Autodesk Fusion 360 part; units mm, degrees
(part 2 of 2)
extrude "Extrude53" add sketch "Sketch37" along normal blind 5.5 contours L0 L1 L2 L3 L4 L5 L6 L7 L9 L10 L11 L12 L13 A5 L16 L18 bodies 2
sketch "Sketch38" plane through (0, 10.5, 0) normal (0, 1, 0) x (-1, 0, 0)
  circle A0 centre (-61.5, 36.5) radius 1.75
  circle A1 centre (-61.5, 5.5) radius 1.75
  line L0 (-56, 21) -> (-56, 42)
  line L1 (-56, 42) -> (-56.125, 42)
  line L2 (-56.125, 42) -> (-56.125, 33.4286)
  line L3 (-56.125, 33.4286) -> (-56.125, 30)
  line L4 (-56.125, 30) -> (-58.125, 30)
  line L5 (-58.125, 30) -> (-58.125, 33.4286)
  line L6 (-58.125, 33.4286) -> (-58.125, 42)
  line L7 (-58.125, 42) -> (-67, 42)
  line L8 (-67, 42) -> (-67, 0)
  line L9 (-67, 0) -> (-25, 0)
  line L10 (-25, 0) -> (-25, 42)
  line L11 (-25, 42) -> (-33.875, 42)
  line L12 (-33.875, 42) -> (-33.875, 33.4286)
  line L13 (-33.875, 33.4286) -> (-33.875, 30)
  line L14 (-33.875, 30) -> (-35.875, 30)
  line L15 (-35.875, 30) -> (-35.875, 33.4286)
  line L16 (-35.875, 33.4286) -> (-35.875, 42)
  line L17 (-35.875, 42) -> (-36, 42)
  line L18 (-36, 42) -> (-36, 21)
  arc A2 (-56, 21) -> (-36, 21) centre (-46, 21) ccw
  circle A3 centre (-30.5, 36.5) radius 1.75
  circle A4 centre (-30.5, 5.5) radius 1.75
  line L19 (-33.875, 30) -> (-35.875, 30)
  line L20 (-35.875, 30) -> (-35.875, 42)
  line L21 (-35.875, 42) -> (-33.875, 42)
  line L22 (-33.875, 42) -> (-33.875, 30)
  line L23 (-56.125, 30) -> (-58.125, 30)
  line L24 (-58.125, 30) -> (-58.125, 42)
  line L25 (-58.125, 42) -> (-56.125, 42)
  line L26 (-56.125, 42) -> (-56.125, 30)
  constraint horizontal L19
  constraint vertical L20
  constraint horizontal L21
  constraint vertical L22
  constraint coincident L16.end L17.start
  constraint coincident L13.end L14.start
  constraint horizontal L23
  constraint vertical L24
  constraint horizontal L25
  constraint vertical L26
  constraint coincident L6.end L7.start
  constraint coincident L3.end L4.start
extrude "Extrude54" add sketch "Sketch38" against normal blind 10.5 contours L2 L3 L4 L5 L6 L23 L24 L25 L26 | L12 L13 L14 L15 L16 L19 L20 L21 L22 bodies 2
sketch "Sketch39" plane through (0, 10.5, 0) normal (0, 1, 0) x (-1, 0, 0)
  circle A0 centre (-61.5, 36.5) radius 1.75
  circle A1 centre (-61.5, 5.5) radius 1.75
  line L0 (-56, 21) -> (-56, 42)
  line L1 (-56, 42) -> (-56.125, 42)
  line L2 (-56.125, 42) -> (-56.125, 33.4286)
  line L3 (-56.125, 33.4286) -> (-58.125, 33.4286)
  line L4 (-58.125, 33.4286) -> (-58.125, 42)
  line L5 (-58.125, 42) -> (-67, 42)
  line L6 (-67, 42) -> (-67, 0)
  line L7 (-67, 0) -> (-25, 0)
  line L8 (-25, 0) -> (-25, 42)
  line L9 (-25, 42) -> (-33.875, 42)
  line L10 (-33.875, 42) -> (-33.875, 33.4286)
  line L11 (-33.875, 33.4286) -> (-35.875, 33.4286)
  line L12 (-35.875, 33.4286) -> (-35.875, 42)
  line L13 (-35.875, 42) -> (-36, 42)
  line L14 (-36, 42) -> (-36, 21)
  arc A2 (-56, 21) -> (-36, 21) centre (-46, 21) ccw
  circle A3 centre (-30.5, 36.5) radius 1.75
  circle A4 centre (-30.5, 5.5) radius 1.75
  circle A5 centre (-46, 21) radius 10.125
  line L15 (-46, 21) -> (-35.875, 21)
  line L16 (-35.875, 21) -> (-56.125, 21)
  line L17 (-56.125, 21) -> (-56.125, 42)
  line L18 (-56.125, 42) -> (-35.875, 42)
  line L19 (-35.875, 42) -> (-35.875, 21)
  dimension "d229" = 20.25
  constraint concentric A2 A5
  constraint coincident A2.centre A5.centre
  constraint coincident A5 L15.end
  constraint perpendicular L14 L15
  constraint horizontal L16
  constraint vertical L17
  constraint horizontal L18
  constraint vertical L19
  constraint coincident L1.end L2.start
  measures "d229" diameter of A5
extrude "Extrude55" cut sketch "Sketch39" against normal blind 5.5 contours L0 A5 L16 | A2 A5 L15 L16 | L0 L1 L2 A5 L17 L18 | L0 L14 A5 L18 | L14 A5 L15 L16 | L12 L13 L14 A5 L18 L19 bodies 2
sketch "Sketch40" plane through (0, 0, 42) normal (0, 0, 1) x (1, 0, 0)
  line L0 (67, 0) -> (67, 10.5)
  line L1 (67, 10.5) -> (58.125, 10.5)
  line L2 (58.125, 10.5) -> (58.125, 0)
  line L3 (58.125, 0) -> (67, 0)
  line L4 (67, 5.25) -> (63.5, 5.25)
  circle A0 centre (63.5, 5.25) radius 1.25
  dimension "d232" = 3.5
  dimension "d233" = 2.5
  constraint midpoint L0 L4.start
  constraint perpendicular L0 L4
  constraint coincident L4.end A0.centre
  measures "d232" distance of L4.start L4.end
  measures "d233" diameter of A0
extrude "Extrude56" cut sketch "Sketch40" against normal blind 3 contours A0 bodies 2
sketch "Sketch41" plane through (0, 0, 42) normal (0, 0, 1) x (1, 0, 0)
  line L0 (25, 0) -> (33.875, 0)
  line L1 (33.875, 0) -> (33.875, 10.5)
  line L2 (33.875, 10.5) -> (25, 10.5)
  line L3 (25, 10.5) -> (25, 0)
  line L4 (25, 5.25) -> (28.5, 5.25)
  circle A0 centre (28.5, 5.25) radius 1.25
  dimension "d236" = 3.5
  dimension "d237" = 2.5
  constraint midpoint L3 L4.start
  constraint perpendicular L3 L4
  constraint coincident L4.end A0.centre
  measures "d236" distance of L4.start L4.end
  measures "d237" diameter of A0
extrude "Extrude57" cut sketch "Sketch41" against normal blind 3 contours A0 bodies 2
sketch "Sketch42" plane through (0, 0, 0) normal (0, 0, -1) x (-1, 0, 0)
  line L0 (-67, 0) -> (-25, 0)
  line L1 (-25, 0) -> (-25, 10.5)
  line L2 (-25, 10.5) -> (-67, 10.5)
  line L3 (-67, 10.5) -> (-67, 0)
  line L4 (-67, 5.25) -> (-63.5, 5.25)
  circle A0 centre (-63.5, 5.25) radius 1.25
  line L5 (-25, 5.25) -> (-28.5, 5.25)
  circle A1 centre (-28.5, 5.25) radius 1.25
  dimension "d240" = 3.5
  dimension "d241" = 2.5
  dimension "d242" = 3.5
  dimension "d243" = 2.5
  constraint midpoint L3 L4.start
  constraint perpendicular L3 L4
  constraint coincident L4.end A0.centre
  constraint midpoint L1 L5.start
  constraint perpendicular L1 L5
  constraint coincident L5.end A1.centre
  measures "d240" distance of L4.start L4.end
  measures "d241" diameter of A0
  measures "d242" distance of L5.start L5.end
  measures "d243" diameter of A1
extrude "Extrude58" cut sketch "Sketch42" against normal blind 3 contours A0 | A1 bodies 2
sketch "Sketch43" plane through (0, 0, 42) normal (0, 0, -1) x (-1, 0, 0)
  line L0 (-35.875, 22.25) -> (-35.875, 24.25)
  line L1 (-35.875, 24.25) -> (-56.125, 24.25)
  line L2 (-56.125, 24.25) -> (-56.125, 22.25)
  line L3 (-56.125, 22.25) -> (-48.5, 22.25)
  line L4 (-48.5, 22.25) -> (-48.5, 15.95)
  line L5 (-48.5, 15.95) -> (-43.5, 15.95)
  line L6 (-43.5, 15.95) -> (-43.5, 22.25)
  line L7 (-43.5, 22.25) -> (-35.875, 22.25)
  line L8 (-48.5, 24.25) -> (-43.5, 24.25)
  line L9 (-43.5, 24.25) -> (-43.5, 5)
  line L10 (-43.5, 5) -> (-48.5, 5)
  line L11 (-48.5, 5) -> (-48.5, 24.25)
  dimension "d246" = 19.25
  constraint horizontal L8
  constraint vertical L9
  constraint horizontal L10
  constraint vertical L11
  constraint coincident L1 L8.start
  measures "d246" distance of L8.start L10.end
extrude "Extrude59" add sketch "Sketch43" along normal blind 5 contours L1 L4 L5 L6 L8 L9 L11 | L5 L9 L10 L11 bodies 2
sketch "Sketch44" plane through (43.5, 0, 0) normal (-1, 0, 0) x (0, 0, 1)
  line L0 (52, 22.25) -> (42, 22.25)
  line L1 (42, 22.25) -> (42, 24.25)
  line L2 (42, 24.25) -> (37, 24.25)
  line L3 (37, 24.25) -> (37, 5)
  line L4 (37, 5) -> (42, 5)
  line L5 (42, 5) -> (42, 2)
  line L6 (42, 2) -> (52, 2)
  line L7 (52, 2) -> (52, 8.34)
  line L8 (52, 8.34) -> (42, 8.34)
  line L9 (42, 8.34) -> (42, 15.95)
  line L10 (42, 15.95) -> (52, 15.95)
  line L11 (52, 15.95) -> (52, 22.25)
  line L12 (42, 24.25) -> (37, 5)
  constraint coincident L1.end L2.start
  constraint coincident L3.end L4.start
extrude "Extrude60" cut sketch "Sketch44" against normal blind 12.625 contours L2 L3 L12 bodies 2
extrude "Extrude61" cut 1 faces at (46.0249, 15.95, 43.3343) along direction (0, 1, 0) blind 0.25 on bodies 2 bodies 2
extrude "Extrude62" add 1 faces at (38.2537, 24.25, 47.0497) along direction (0, 1, 0) blind 0.5 on bodies 2 bodies 2
extrude "Extrude63" cut 1 faces at (40.9583, 22.25, 45.3333) along direction (0, 1, 0) blind 0.25 on bodies 2 bodies 2
extrude "Extrude64" cut 1 faces at (51.0417, 22.25, 45.3333) along direction (0, 1, 0) blind 0.25 on bodies 2 bodies 2
extrude "Extrude65" cut 1 faces at (48.5, 5.1133, 48.6667) along direction (-1, 0, 0) blind 0.125 on bodies 2 bodies 2
extrude "Extrude66" cut 1 faces at (43.5, 5.1133, 48.6667) along direction (1, 0, 0) blind 0.125 on bodies 2 bodies 2
sketch "Sketch45" plane through (43.625, 0, 0) normal (-1, 0, 0) x (0, 0, 1)
  line L0 (42, 16.2) -> (52, 16.2)
  line L1 (52, 16.2) -> (52, 22.5)
  line L2 (52, 22.5) -> (42, 22.5)
  line L3 (42, 22.5) -> (42, 24.25)
  line L4 (42, 24.25) -> (37, 5)
  line L5 (37, 5) -> (42, 5)
  line L6 (42, 5) -> (42, 2)
  line L7 (42, 2) -> (52, 2)
  line L8 (52, 2) -> (52, 8.34)
  line L9 (52, 8.34) -> (42, 8.34)
  line L10 (42, 8.34) -> (42, 16.2)
  line L11 (42, 24.25) -> (42, 24.75)
  line L12 (42, 24.75) -> (33, 5)
  line L13 (33, 5) -> (37, 5)
  constraint coincident L3.end L4.start
  constraint parallel L3 L11
  constraint coincident L4.end L5.start
extrude "Extrude67" add sketch "Sketch45" against normal blind 4.75 contours L4 L11 L12 L13 bodies 2
extrude "Extrude68" cut 1 faces at (45.7478, 10.5, 6.5076) along direction (0, -1, 0) blind 10.5 on bodies 2 bodies 2
sketch "Sketch46" plane through (0, 5, 0) normal (0, 1, 0) x (-1, 0, 0)
  line L0 (-48.375, 33) -> (-48.375, 42)
  line L1 (-48.375, 42) -> (-56.125, 42)
  line L2 (-56.125, 42) -> (-56.125, 33.4286)
  line L3 (-56.125, 33.4286) -> (-56.125, 21)
  arc A0 (-56.125, 21) -> (-35.875, 21) centre (-46, 21) ccw
  line L4 (-35.875, 21) -> (-35.875, 33.4286)
  line L5 (-35.875, 33.4286) -> (-35.875, 42)
  line L6 (-35.875, 42) -> (-43.625, 42)
  line L7 (-43.625, 42) -> (-43.625, 33)
  line L8 (-43.625, 33) -> (-48.375, 33)
  circle A1 centre (-46, 21) radius 8.625
  line L9 (-34, 42) -> (-61, 42)
  line L10 (-61, 42) -> (-61, 10)
  line L11 (-61, 10) -> (-34, 10)
  line L12 (-34, 10) -> (-34, 42)
  constraint horizontal L9
  constraint vertical L10
  constraint horizontal L11
  constraint vertical L12
extrude "Extrude69" cut sketch "Sketch46" along normal blind 41 and the other way blind 18 bodies 2
sketch "Sketch47" plane through (33.875, 0, 0) normal (-1, 0, 0) x (0, 0, 1)
  line L0 (33.4286, 10.5) -> (33.4286, 0)
  line L1 (33.4286, 0) -> (52, 0)
  line L2 (52, 0) -> (52, 24.75)
  line L3 (52, 24.75) -> (42, 24.75)
  line L4 (42, 24.75) -> (42, 24.25)
  line L5 (42, 24.25) -> (33.4286, 10.5)
  line L6 (42, 0) -> (42, 24.75)
  line L7 (42, 0) -> (27, 0)
  line L8 (27, 0) -> (27, 26)
  line L9 (27, 26) -> (42, 26)
  line L10 (42, 26) -> (42, 0)
  constraint coincident L1 L6.start
  constraint coincident L3.end L4.start
  constraint horizontal L7
  constraint vertical L8
  constraint horizontal L9
  constraint vertical L10
extrude "Extrude70" cut sketch "Sketch47" against normal blind 10 contours L0 L1 L5 L6 L7 L10 bodies 2
sketch "Sketch48" plane through (0, 0, 42) normal (0, 0, -1) x (-1, 0, 0)
  line L0 (-33.875, 0) -> (-33.875, 24.75)
  line L1 (-33.875, 24.75) -> (-58.125, 24.75)
  line L2 (-58.125, 24.75) -> (-58.125, 0)
  line L3 (-58.125, 0) -> (-33.875, 0)
  line L4 (-48.375, 16.2) -> (-43.625, 16.2)
  line L5 (-43.625, 16.2) -> (-43.625, 22.5)
  line L6 (-43.625, 22.5) -> (-35.875, 22.5)
  line L7 (-35.875, 22.5) -> (-35.875, 2)
  line L8 (-35.875, 2) -> (-43.625, 2)
  line L9 (-43.625, 2) -> (-43.625, 8.34)
  line L10 (-43.625, 8.34) -> (-48.375, 8.34)
  line L11 (-48.375, 8.34) -> (-48.375, 2)
  line L12 (-48.375, 2) -> (-56.125, 2)
  line L13 (-56.125, 2) -> (-56.125, 22.5)
  line L14 (-56.125, 22.5) -> (-48.375, 22.5)
  line L15 (-48.375, 22.5) -> (-48.375, 16.2)
  line L16 (-56.125, 22.5) -> (-56.125, 19)
  line L17 (-56.125, 19) -> (-35.875, 19)
  line L18 (-56.125, 2) -> (-56.125, 5.5)
  line L19 (-56.125, 5.5) -> (-35.875, 5.5)
  line L20 (-56.125, 19) -> (-55, 19)
  line L21 (-55, 19) -> (-55, 5.5)
  line L22 (-35.875, 5.5) -> (-37, 5.5)
  line L23 (-37, 5.5) -> (-37, 19)
  constraint coincident L13.end L14.start
  constraint coincident L13 L16.end
  constraint perpendicular L14 L16
  constraint coincident L7 L17.end
  constraint perpendicular L7 L17
  constraint coincident L12.end L13.start
  constraint coincident L13 L18.end
  constraint perpendicular L12 L18
  constraint coincident L7 L19.end
  constraint perpendicular L7 L19
  constraint coincident L17 L20.end
  constraint perpendicular L16 L20
  constraint coincident L19 L21.end
  constraint perpendicular L19 L21
  constraint coincident L19 L22.end
  constraint perpendicular L7 L22
  constraint coincident L17 L23.end
  constraint perpendicular L17 L23
extrude "Extrude71" add sketch "Sketch48" along normal blind 20 contours L0 L1 L2 L3 | L13 L14 L15 L16 L17 L20 | L5 L6 L7 L17 | L13 L17 L19 L20 L21 | L7 L17 L19 L22 L23 | L11 L12 L13 L18 L19 | L7 L8 L9 L19 L22 bodies 2
extrude "Extrude72" add 1 faces at (45.9751, 8.34, 43.3343) along direction (0, 1, 0) blind 0.1 on bodies 2 bodies 2
extrude "Extrude73" cut 1 faces at (46.0249, 16.2, 43.3343) along direction (0, 1, 0) blind 0.1 on bodies 2 bodies 2
sketch "Sketch49" plane through (0, 19, 0) normal (0, -1, 0) x (1, 0, 0)
  line L0 (55, 42) -> (48.375, 42)
  line L1 (48.375, 42) -> (43.625, 42)
  line L2 (43.625, 42) -> (37, 42)
  line L3 (37, 42) -> (37, 22)
  line L4 (37, 22) -> (55, 22)
  line L5 (55, 22) -> (55, 42)
  line L6 (46, 42) -> (46, 32)
  circle A0 centre (46, 32) radius 3.5
  dimension "d279" = 7
  constraint midpoint L1 L6.start
  constraint perpendicular L4 L6
  constraint coincident L6.end A0.centre
  measures "d279" diameter of A0
extrude "Extrude74" add sketch "Sketch49" along normal blind 2.5 contours A0 bodies 2
sketch "Sketch50" plane through (0, 5.5, 0) normal (0, 1, 0) x (-1, 0, 0)
  line L0 (-37, 42) -> (-43.625, 42)
  line L1 (-43.625, 42) -> (-48.375, 42)
  line L2 (-48.375, 42) -> (-55, 42)
  line L3 (-55, 42) -> (-55, 22)
  line L4 (-55, 22) -> (-37, 22)
  line L5 (-37, 22) -> (-37, 42)
  line L6 (-46, 42) -> (-46, 32)
  circle A0 centre (-46, 32) radius 3.5
  dimension "d282" = 7
  constraint midpoint L1 L6.start
  constraint perpendicular L1 L6
  constraint coincident L6.end A0.centre
  measures "d282" diameter of A0
extrude "Extrude75" add sketch "Sketch50" along normal blind 2.5 contours A0 bodies 2
sketch "Sketch51" plane through (0, 8, 0) normal (0, 1, 0) x (-1, 0, 0)
  circle A0 centre (-46, 32) radius 3.5
  circle A1 centre (-46, 32) radius 1.5
  dimension "d285" = 3
  constraint concentric A0 A1
  measures "d285" diameter of A1
extrude "Extrude76" cut sketch "Sketch51" along normal blind 22 and the other way blind 13 contours A1 bodies 2
sketch "Sketch52" plane through (0, 8.44, 0) normal (0, 1, 0) x (-1, 0, 0)
  line L0 (-43.625, 42) -> (-43.625, 52)
  line L1 (-43.625, 52) -> (-48.375, 52)
  line L2 (-48.375, 52) -> (-48.375, 42)
  line L3 (-48.375, 42) -> (-43.625, 42)
  circle A0 centre (-46, 47) radius 1
  circle A1 centre (-46, 47) radius 1
  constraint concentric A0 A1
extrude "Extrude77" add sketch "Sketch52" against normal blind 8.44 contours A0 A1 bodies 2
sketch "Sketch53" plane through (0, 16.3, 0) normal (0, -1, 0) x (1, 0, 0)
  circle A0 centre (46, 47) radius 1
  line L0 (43.625, 52) -> (43.625, 42)
  line L1 (43.625, 42) -> (48.375, 42)
  line L2 (48.375, 42) -> (48.375, 52)
  line L3 (48.375, 52) -> (43.625, 52)
  circle A1 centre (46, 47) radius 1
  constraint concentric A0 A1
extrude "Extrude78" add sketch "Sketch53" against normal blind 8.45 contours A0 A1 bodies 2
sketch "Sketch54" plane through (0, 24.75, 0) normal (0, 1, 0) x (-1, 0, 0)
  circle A0 centre (-46, 32) radius 1.5
  line L0 (-33.875, 42) -> (-33.875, 52)
  line L1 (-33.875, 52) -> (-58.125, 52)
  line L2 (-58.125, 52) -> (-58.125, 42)
  line L3 (-58.125, 42) -> (-58.125, 22)
  line L4 (-58.125, 22) -> (-33.875, 22)
  line L5 (-33.875, 22) -> (-33.875, 42)
  circle A1 centre (-46, 32) radius 12.125
  constraint concentric A0 A1
  constraint tangent L3 A1
extrude "Extrude79" cut sketch "Sketch54" against normal blind 41 contours L4 L5 A1 | L3 L4 A1 bodies 2
sketch "Sketch55" plane through (0, 24.75, 0) normal (0, 1, 0) x (-1, 0, 0)
  circle A0 centre (-46, 32) radius 1.5
  arc A1 (-39.1432, 22) -> (-33.875, 32) centre (-46, 32) ccw
  line L0 (-33.875, 32) -> (-33.875, 42)
  line L1 (-33.875, 42) -> (-33.875, 52)
  line L2 (-33.875, 52) -> (-58.125, 52)
  line L3 (-58.125, 52) -> (-58.125, 42)
  line L4 (-58.125, 42) -> (-58.125, 32)
  arc A2 (-58.125, 32) -> (-52.8568, 22) centre (-46, 32) ccw
  line L5 (-52.8568, 22) -> (-39.1432, 22)
extrude "Extrude80" cut 1 faces at (56.125, 15.6667, 45.3333) along direction (1, 0, 0) blind 0.125 on bodies 2 bodies 2
extrude "Extrude81" cut 1 faces at (56.25, 15.6667, 45.3333) along direction (1, 0, 0) blind 0.125 on bodies 2 bodies 2
extrude "Extrude82" cut 1 faces at (35.875, 9.8333, 48.6667) along direction (-1, 0, 0) blind 0.25 on bodies 2 bodies 2
extrude "Extrude83" cut 1 faces at (43.1853, 8, 32.2484) along direction (0, -1, 0) blind 0.25 on bodies 2 bodies 2
extrude "Extrude84" cut 1 faces at (45.2029, 16.5, 34.7109) along direction (0, 1, 0) blind 0.25 on bodies 2 bodies 2
extrude "Extrude85" cut 1 faces at (45.2029, 16.75, 34.7109) along direction (0, 1, 0) blind 0.125 on bodies 2 bodies 2
extrude "Extrude86" cut 1 faces at (43.1853, 7.75, 32.2484) along direction (0, -1, 0) blind 0.125 on bodies 2 bodies 2
sketch "Sketch56" plane through (0, 0, 42) normal (0, 0, 1) x (1, 0, 0)
  line L0 (48.375, 22.5) -> (48.375, 19)
  line L1 (48.375, 19) -> (55, 19)
  line L2 (55, 19) -> (55, 5.5)
  line L3 (55, 5.5) -> (48.375, 5.5)
  line L4 (48.375, 5.5) -> (48.375, 2)
  line L5 (48.375, 2) -> (56.375, 2)
  line L6 (56.375, 2) -> (56.375, 22.5)
  line L7 (56.375, 22.5) -> (48.375, 22.5)
  line L8 (55, 19) -> (56, 19)
  line L9 (56, 19) -> (56, 5.5)
  line L10 (56, 5.5) -> (55, 5.5)
  line L11 (55, 5.5) -> (55, 19)
  line L12 (37, 5.5) -> (36, 5.5)
  line L13 (36, 5.5) -> (36, 19)
  line L14 (36, 19) -> (37, 19)
  line L15 (37, 19) -> (37, 5.5)
  dimension "d310" = 1
  dimension "d311" = 1
  dimension "d312" = 13.5
  constraint horizontal L8
  constraint vertical L9
  constraint horizontal L10
  constraint vertical L11
  constraint coincident L1.end L2.start
  constraint horizontal L12
  constraint vertical L13
  constraint horizontal L14
  constraint vertical L15
  measures "d310" distance of L1.end L8.end
  measures "d311" distance of L12.start L12.end
  measures "d312" distance of L12.start L14.end
extrude "Extrude87" cut sketch "Sketch56" against normal blind 29 contours L2 L8 L9 L10 L11 | L12 L13 L14 L15 bodies 2
extrude "Extrude88" add 1 faces at (46.7917, 4.1467, 52) along direction (0, 0, 1) blind 11 on bodies 2 bodies 2
extrude "Extrude89" add 1 faces at (53.5833, 3.1667, 42) along direction (0, 0, 1) blind 11 on bodies 2 bodies 2
extrude "Extrude90" add 1 faces at (38.75, 21.3333, 42) along direction (0, 0, 1) blind 11 on bodies 2 bodies 2
hidden bodies 1
